Autodesk Inventor part; units mm, degrees
(part 2 of 3)
sketch "Sketch6" plane through (0, 6405, 0) normal (0, 1, 0) x (1, 0, 0)
  line L0 (350, -424.749) -> (350, 440.76)
  arc A0 (24.4727, -474.749) -> (24.4727, -424.749) centre (24.4727, -449.749) ccw
  arc A1 (-24.4727, -424.749) -> (-24.4727, -474.749) centre (-24.4727, -449.749) ccw
  line L1 (-350, -424.749) -> (-350, 440.76)
  line L2 (335.0195, -474.749) -> (364.9805, -474.749)
  line L3 (335.0195, -424.749) -> (364.9805, -424.749)
  arc A2 (364.9805, -474.749) -> (364.9805, -424.749) centre (364.9805, -449.749) ccw
  arc A3 (335.0195, -424.749) -> (335.0195, -474.749) centre (335.0195, -449.749) ccw
  line L4 (0, -424.749) -> (0, 440.76)
  line L5 (-24.4727, -474.749) -> (24.4727, -474.749)
  line L6 (-24.4727, -424.749) -> (24.4727, -424.749)
  line L7 (-364.9805, -474.749) -> (-335.0195, -474.749)
  line L8 (-489.5054, 350) -> (407.7236, 350)
  line L9 (-544.4663, 325) -> (-514.5054, 325)
  line L10 (-544.4663, 375) -> (-514.5054, 375)
  arc A4 (-514.5054, 325) -> (-514.5054, 375) centre (-514.5054, 350) ccw
  arc A5 (-544.4663, 375) -> (-544.4663, 325) centre (-544.4663, 350) ccw
  line L11 (-489.5054, 0) -> (-476.6036, 0)
  line L12 (-441.6036, 0) -> (407.7236, 0)
  line L13 (-559.9204, -25) -> (-514.5054, -25)
  line L14 (-559.9204, 25) -> (-514.5054, 25)
  arc A6 (-514.5054, -25) -> (-514.5054, 25) centre (-514.5054, 0) ccw
  line L15 (-364.9805, -424.749) -> (-335.0195, -424.749)
  arc A7 (-335.0195, -474.749) -> (-335.0195, -424.749) centre (-335.0195, -449.749) ccw
  arc A8 (-364.9805, -424.749) -> (-364.9805, -474.749) centre (-364.9805, -449.749) ccw
  line L16 (-489.5054, -350) -> (407.7236, -350)
  line L17 (-544.4663, -375) -> (-514.5054, -375)
  line L18 (-544.4663, -325) -> (-514.5054, -325)
  arc A9 (-514.5054, -375) -> (-514.5054, -325) centre (-514.5054, -350) ccw
  arc A10 (-544.4663, -325) -> (-544.4663, -375) centre (-544.4663, -350) ccw
  line L19 (145.0003, 447.2664) -> (120.0003, 442.2664)
  line L20 (120.0003, 130.0003) -> (120.0003, 467.2664)
  line L21 (120.0003, 442.2664) -> (350, 442.2664)
  line L22 (-439.1036, 145.0003) -> (-429.1036, 145.0003)
  line L23 (-429.1036, 145.0003) -> (-434.1036, 120.0003)
  line L24 (-439.1036, 145.0003) -> (-434.1036, 120.0003)
  line L25 (-130.0003, 120.0003) -> (-459.1036, 120.0003)
  line L26 (-434.1036, 120.0003) -> (-434.1036, 350)
  line L27 (-145.0003, 437.2664) -> (-145.0003, 447.2664)
  line L28 (-145.0003, 447.2664) -> (-120.0003, 442.2664)
  line L29 (-145.0003, 437.2664) -> (-120.0003, 442.2664)
  line L30 (-120.0003, 130.0003) -> (-120.0003, 467.2664)
  line L31 (-325, 447.2664) -> (-325, 437.2664)
  line L32 (-325, 437.2664) -> (-350, 442.2664)
  line L33 (-325, 447.2664) -> (-350, 442.2664)
  line L34 (-439.1036, -95.0003) -> (-434.1036, -120.0003)
  line L35 (-350, 360) -> (-350, 467.2664)
  line L36 (-350, 442.2664) -> (-120.0003, 442.2664)
  line L37 (95.0003, 437.2664) -> (95.0003, 447.2664)
  line L38 (95.0003, 447.2664) -> (120.0003, 442.2664)
  line L39 (95.0003, 437.2664) -> (120.0003, 442.2664)
  line L40 (120.0003, 130.0003) -> (120.0003, 467.2664)
  line L41 (-95.0003, 447.2664) -> (-95.0003, 437.2664)
  line L42 (-95.0003, 437.2664) -> (-120.0003, 442.2664)
  line L43 (-95.0003, 447.2664) -> (-120.0003, 442.2664)
  line L44 (-120.0003, 130.0003) -> (-120.0003, 467.2664)
  line L45 (-120.0003, 442.2664) -> (120.0003, 442.2664)
  line L46 (325, 437.2664) -> (325, 447.2664)
  line L47 (325, 447.2664) -> (350, 442.2664)
  line L48 (325, 437.2664) -> (350, 442.2664)
  line L49 (350, 360) -> (350, 467.2664)
  line L50 (145.0003, 447.2664) -> (145.0003, 437.2664)
  line L51 (145.0003, 437.2664) -> (120.0003, 442.2664)
  line L52 (350, 442.2664) -> (646.147, 442.2664)
  line L53 (-360, 350) -> (-459.1036, 350)
  line L54 (-429.1036, 325) -> (-434.1036, 350)
  line L55 (-439.1036, 325) -> (-434.1036, 350)
  line L56 (-429.1036, 325) -> (-439.1036, 325)
  line L57 (-434.1036, -120.0003) -> (-434.1036, 120.0003)
  line L58 (-130.0003, -120.0003) -> (-459.1036, -120.0003)
  line L59 (-429.1036, -95.0003) -> (-434.1036, -120.0003)
  line L60 (-439.1036, -95.0003) -> (-429.1036, -95.0003)
  line L61 (-130.0003, 120.0003) -> (-459.1036, 120.0003)
  line L62 (-429.1036, 95.0003) -> (-434.1036, 120.0003)
  line L63 (-439.1036, 95.0003) -> (-434.1036, 120.0003)
  line L64 (-429.1036, 95.0003) -> (-439.1036, 95.0003)
  line L65 (-434.1036, -350) -> (-434.1036, -120.0003)
  line L66 (-360, -350) -> (-459.1036, -350)
  line L67 (-439.1036, -325) -> (-434.1036, -350)
  line L68 (-429.1036, -325) -> (-434.1036, -350)
  line L69 (-439.1036, -325) -> (-429.1036, -325)
  line L70 (-130.0003, -120.0003) -> (-459.1036, -120.0003)
  line L71 (-429.1036, -145.0003) -> (-434.1036, -120.0003)
  line L72 (-439.1036, -145.0003) -> (-434.1036, -120.0003)
  line L73 (-429.1036, -145.0003) -> (-439.1036, -145.0003)
  line L74 (-350, 310) -> (-350, 350)
  line L75 (-342, 318) -> (-342, 332)
  line L76 (-318, 342) -> (-332, 342)
  line L77 (-310, 350) -> (-350, 350)
  line L78 (-342, 332) -> (-341.2388, 335.8268)
  arc A11 (-335.8268, 341.2388) -> (-341.2388, 335.8268) centre (-332, 332) ccw
  line L79 (-335.8268, 341.2388) -> (-332, 342)
  line L80 (-318, -342) -> (-332, -342)
  line L81 (-342, -332) -> (-342, -318)
  line L82 (-350, -350) -> (-350, -310)
  line L83 (-310, -350) -> (-350, -350)
  line L84 (-332, -342) -> (-335.8268, -341.2388)
  arc A12 (-341.2388, -335.8268) -> (-335.8268, -341.2388) centre (-332, -332) ccw
  line L85 (-341.2388, -335.8268) -> (-342, -332)
  line L86 (350, -350) -> (350, -310)
  line L87 (342, -332) -> (342, -318)
  line L88 (332, -342) -> (318, -342)
  line L89 (350, -350) -> (310, -350)
  line L90 (342, -332) -> (341.2388, -335.8268)
  arc A13 (335.8268, -341.2388) -> (341.2388, -335.8268) centre (332, -332) ccw
  line L91 (335.8268, -341.2388) -> (332, -342)
  circle A14 centre (-120, -120) radius 9
  line L92 (-102, -120) -> (-138, -120)
  line L93 (-120, -102) -> (-120, -138)
  circle A15 centre (120, -120) radius 9
  line L94 (138, -120) -> (102, -120)
  line L95 (120, -102) -> (120, -138)
  circle A16 centre (-120, 120) radius 9
  line L96 (-102, 120) -> (-138, 120)
  line L97 (-120, 138) -> (-120, 102)
  circle A17 centre (120, 120) radius 9
  line L98 (138, 120) -> (102, 120)
  line L99 (120, 138) -> (120, 102)
  line L100 (-354, 0) -> (-342, 0)
  line L101 (-350, 4) -> (-342, 4)
  line L102 (-350, -4) -> (-342, -4)
  line L103 (350, 310) -> (310, 350)
  line L104 (310, 350) -> (-310, 350)
  line L105 (350, 310) -> (350, -310)
  line L106 (350, -310) -> (310, -350)
  line L107 (-310, -350) -> (-350, -310)
  line L108 (-350, -310) -> (-350, 310)
  line L109 (-350, 310) -> (-310, 350)
  line L110 (310, -350) -> (-310, -350)
  line L111 (332, 342) -> (318, 342)
  line L112 (342, 318) -> (342, 332)
  line L113 (350, 310) -> (350, 350)
  line L114 (350, 350) -> (310, 350)
  line L115 (332, 342) -> (335.8268, 341.2388)
  arc A18 (341.2388, 335.8268) -> (335.8268, 341.2388) centre (332, 332) ccw
  line L116 (341.2388, 335.8268) -> (342, 332)
  line L117 (-347, 270) -> (-345.0866, 270.3806)
  line L118 (273.0866, -342.3806) -> (271.4645, -343.4645)
  line L119 (271.4645, -343.4645) -> (270.3806, -345.0866)
  line L120 (-270.3806, 345.0866) -> (-270, 347)
  line L121 (-271.4645, 343.4645) -> (-270.3806, 345.0866)
  line L122 (-273.0866, 342.3806) -> (-271.4645, 343.4645)
  line L123 (-275, 342) -> (-273.0866, 342.3806)
  line L124 (-342.3806, 273.0866) -> (-342, 275)
  line L125 (-343.4645, 271.4645) -> (-342.3806, 273.0866)
  line L126 (-345.0866, 270.3806) -> (-343.4645, 271.4645)
  line L127 (342, 275) -> (342.3806, 273.0866)
  line L128 (-270, 350) -> (-310, 350)
  line L129 (-270, 347) -> (-270, 350)
  line L130 (-275, 342) -> (-318, 342)
  line L131 (-342, 275) -> (-342, 318)
  line L132 (-350, 270) -> (-347, 270)
  line L133 (-350, 270) -> (-350, 310)
  line L134 (345.0866, 270.3806) -> (347, 270)
  line L135 (343.4645, 271.4645) -> (345.0866, 270.3806)
  line L136 (342.3806, 273.0866) -> (343.4645, 271.4645)
  line L137 (270.3806, -345.0866) -> (270, -347)
  line L138 (273.0866, 342.3806) -> (275, 342)
  line L139 (271.4645, 343.4645) -> (273.0866, 342.3806)
  line L140 (270.3806, 345.0866) -> (271.4645, 343.4645)
  line L141 (270, 347) -> (270.3806, 345.0866)
  line L142 (310, 350) -> (270, 350)
  line L143 (350, 270) -> (350, 310)
  line L144 (347, 270) -> (350, 270)
  line L145 (342, 275) -> (342, 318)
  line L146 (318, 342) -> (275, 342)
  line L147 (270, 347) -> (270, 350)
  line L148 (342, 270) -> (350, 270)
  line L149 (342, -270) -> (342, 270)
  line L150 (350, -270) -> (342, -270)
  line L151 (270, 342) -> (270, 350)
  line L152 (-270, 342) -> (270, 342)
  line L153 (-270, 350) -> (-270, 342)
  line L154 (270, 350) -> (-270, 350)
  line L155 (-342, 270) -> (-350, 270)
  line L156 (-342, -270) -> (-342, 270)
  line L157 (-350, -270) -> (-342, -270)
  line L158 (-350, 270) -> (-350, -270)
  line L159 (-270, -342) -> (270, -342)
  line L160 (-270, -350) -> (-270, -342)
  line L161 (270, -350) -> (270, -342)
  line L162 (-270, -350) -> (270, -350)
  line L163 (-270.3806, -345.0866) -> (-271.4645, -343.4645)
  line L164 (-271.4645, -343.4645) -> (-273.0866, -342.3806)
  line L165 (-273.0866, -342.3806) -> (-275, -342)
  line L166 (-342, -275) -> (-342.3806, -273.0866)
  line L167 (-342.3806, -273.0866) -> (-343.4645, -271.4645)
  line L168 (-343.4645, -271.4645) -> (-345.0866, -270.3806)
  line L169 (-345.0866, -270.3806) -> (-347, -270)
  line L170 (-270, -350) -> (-270, -347)
  line L171 (-275, -342) -> (-318, -342)
  line L172 (350, 270) -> (350, -270)
  line L173 (-342, -318) -> (-342, -275)
  line L174 (-350, -270) -> (-347, -270)
  line L175 (-350, -310) -> (-350, -270)
  line L176 (-270, -350) -> (-310, -350)
  line L177 (-270, -347) -> (-270.3806, -345.0866)
  line L178 (350, -310) -> (350, -270)
  line L179 (350, -270) -> (347, -270)
  line L180 (342, -318) -> (342, -275)
  line L181 (318, -342) -> (275, -342)
  line L182 (270, -350) -> (270, -347)
  line L183 (310, -350) -> (270, -350)
  line L184 (347, -270) -> (345.0866, -270.3806)
  line L185 (345.0866, -270.3806) -> (343.4645, -271.4645)
  line L186 (343.4645, -271.4645) -> (342.3806, -273.0866)
  line L187 (342.3806, -273.0866) -> (342, -275)
  line L188 (275, -342) -> (273.0866, -342.3806)
  line L189 (379.0739, 240.3123) -> (409.0739, 240.3123)
  line L190 (409.0739, 215.6456) -> (605.1413, 215.6456)
  line L191 (409.0739, 252.6456) -> (605.1413, 252.6456)
  line L192 (605.1413, 215.6456) -> (605.1413, 252.6456)
  line L193 (409.0739, 215.6456) -> (409.0739, 252.6456)
  line L194 (120, 120) -> (379.0739, 240.3123)
  line L195 (-58.2993, 546.2236) -> (67.1733, 546.2236)
  point P0 (0, 0)
  point P1 (-354.9805, -464.749)
  point P2 (-14.4727, -464.749)
  point P3 (345.0195, -464.749)
  point P4 (-534.4663, 335)
  point P5 (-549.9204, -15)
  point P6 (-534.4663, -365)
  point P7 (-262.8139, 454.7664)
  point P8 (375, 454.7664)
  point P9 (-27.8137, 454.7664)
  point P10 (207.1864, 454.7664)
  point P11 (-446.6036, 207.1864)
  point P12 (-446.6036, -27.8137)
  point P13 (-446.6036, -262.8139)
  point P14 (415.0739, 221.6456)
  point P15 (442.9231, 221.6456)
  point P16 (537.1784, 221.6456)
  point P17 (21.5405, 553.7236)
  point P18 (-25.7205, 513.7236)
  point P19 (-12.6665, 553.7236)
  point P20 (-58.2993, 553.7236)
  constraints: 384 end point, 47 point on line, 33 point on circle, 19 centre point, 4 midpoint, 66 other
sketch "Sketch7" plane through (0, 6405, 0) normal (0, 1, 0) x (1, 0, 0)
  line L0 (-350, -350) -> (-270, -350) projected
  line L1 (-310, -350) -> (-350, -310)
  line L2 (-350, -270) -> (-350, -350) projected
  line L3 (-350, -310) -> (-350, 310)
  line L4 (-350, 350) -> (-350, 270) projected
  line L5 (-350, 310) -> (-310, 350)
  line L6 (-310, 350) -> (310, 350)
  line L7 (310, 350) -> (350, 310)
  line L8 (350, 310) -> (350, -310)
  line L9 (350, -310) -> (310, -350)
  line L10 (310, -350) -> (-310, -350)
  circle A0 centre (-120, -120) radius 9 projected
  circle A1 centre (120, -120) radius 9 projected
  circle A2 centre (120, 120) radius 9 projected
  circle A3 centre (-120, 120) radius 9 projected
  point P0 (0, 0)
  constraints: 16 end point, 4 perpendicular, 3 midpoint, 1 collinear, 1 parallel
extrude "Extrusion17" add sketch "Sketch7" along normal blind 10 separate body contours L1 L2 L3 L5 L6 L7 L8 L9 L10 L0
sketch "Sketch8" plane through (-270, 15, 350) normal (0, 0, 1) x (1, 0, 0)
  arc A0 (33330.0195, 14726.87) -> (33330.0195, 14676.87) centre (33330.0195, 14701.87) ccw
  arc A1 (34059.9805, 14676.87) -> (34059.9805, 14726.87) centre (34059.9805, 14701.87) ccw
  arc A2 (34030.0195, 14726.87) -> (34030.0195, 14676.87) centre (34030.0195, 14701.87) ccw
  line L0 (33695, 14726.87) -> (33695, 15412.2236)
  line L1 (33695, 15461.2236) -> (33695, 21400.56)
  line L2 (33672.2925, 14676.87) -> (33717.7075, 14676.87)
  line L3 (33672.2925, 14726.87) -> (33717.7075, 14726.87)
  arc A3 (33717.7075, 14676.87) -> (33717.7075, 14726.87) centre (33717.7075, 14701.87) ccw
  arc A4 (33672.2925, 14726.87) -> (33672.2925, 14676.87) centre (33672.2925, 14701.87) ccw
  line L4 (33345, 14726.87) -> (33345, 21400.56)
  line L5 (33330.0195, 14676.87) -> (33359.9805, 14676.87)
  line L6 (33187.65, 14882.4) -> (34188.23, 14882.4)
  line L7 (33040.2135, 14857.4) -> (33162.65, 14857.4)
  line L8 (33040.2135, 14907.4) -> (33162.65, 14907.4)
  arc A5 (33162.65, 14857.4) -> (33162.65, 14907.4) centre (33162.65, 14882.4) ccw
  line L9 (33330.0195, 14726.87) -> (33359.9805, 14726.87)
  arc A6 (33040.2135, 14907.4) -> (33040.2135, 14857.4) centre (33040.2135, 14882.4) ccw
  line L10 (34045, 14726.87) -> (34045, 15229.9)
  line L11 (33187.65, 21282.4) -> (34188.23, 21282.4)
  line L12 (34045, 15264.9) -> (34045, 21400.56)
  line L13 (34030.0195, 14676.87) -> (34059.9805, 14676.87)
  line L14 (34030.0195, 14726.87) -> (34059.9805, 14726.87)
  line L15 (33025.7555, 21257.4) -> (33162.65, 21257.4)
  line L16 (33025.7555, 21307.4) -> (33162.65, 21307.4)
  arc A7 (33162.65, 21257.4) -> (33162.65, 21307.4) centre (33162.65, 21282.4) ccw
  arc A8 (33025.7555, 21307.4) -> (33025.7555, 21257.4) centre (33025.7555, 21282.4) ccw
  arc A9 (33359.9805, 14676.87) -> (33359.9805, 14726.87) centre (33359.9805, 14701.87) ccw
  arc A10 (34483.8578, 21307.4) -> (34483.8578, 21257.4) centre (34483.8578, 21282.4) ccw
  arc A11 (34498.3158, 14907.4) -> (34498.3158, 14857.4) centre (34498.3158, 14882.4) ccw
  line L17 (34320.5776, 17577.4) -> (34310.5776, 17577.4)
  line L18 (34310.5776, 17577.4) -> (34315.5776, 17602.4)
  line L19 (34320.5776, 17577.4) -> (34315.5776, 17602.4)
  line L20 (34315.5776, 19702.4) -> (34315.5776, 20052.4)
  line L21 (34320.5776, 16177.4) -> (34310.5776, 16177.4)
  line L22 (34310.5776, 16177.4) -> (34315.5776, 16202.4)
  line L23 (34320.5776, 16177.4) -> (34315.5776, 16202.4)
  line L24 (34015, 16202.4) -> (34335.5776, 16202.4)
  line L25 (34320.5776, 19677.4) -> (34310.5776, 19677.4)
  line L26 (34310.5776, 19677.4) -> (34315.5776, 19702.4)
  line L27 (34320.5776, 19677.4) -> (34315.5776, 19702.4)
  line L28 (34015, 19702.4) -> (34335.5776, 19702.4)
  line L29 (34310.5776, 19377.4) -> (34320.5776, 19377.4)
  line L30 (34320.5776, 19377.4) -> (34315.5776, 19352.4)
  line L31 (34015, 17602.4) -> (34335.5776, 17602.4)
  line L32 (34310.5776, 17277.4) -> (34320.5776, 17277.4)
  line L33 (34320.5776, 17277.4) -> (34315.5776, 17252.4)
  line L34 (34310.5776, 17277.4) -> (34315.5776, 17252.4)
  line L35 (34310.5776, 19377.4) -> (34315.5776, 19352.4)
  line L36 (34015, 19352.4) -> (34335.5776, 19352.4)
  line L37 (34315.5776, 19352.4) -> (34315.5776, 19702.4)
  line L38 (34320.5776, 19327.4) -> (34310.5776, 19327.4)
  line L39 (34310.5776, 19327.4) -> (34315.5776, 19352.4)
  line L40 (34015, 17252.4) -> (34335.5776, 17252.4)
  line L41 (34310.5776, 15877.4) -> (34320.5776, 15877.4)
  line L42 (34320.5776, 15877.4) -> (34315.5776, 15852.4)
  line L43 (34310.5776, 15877.4) -> (34315.5776, 15852.4)
  line L44 (34320.5776, 19327.4) -> (34315.5776, 19352.4)
  line L45 (34015, 19352.4) -> (34335.5776, 19352.4)
  line L46 (34310.5776, 19027.4) -> (34320.5776, 19027.4)
  line L47 (34320.5776, 19027.4) -> (34315.5776, 19002.4)
  line L48 (34310.5776, 19027.4) -> (34315.5776, 19002.4)
  line L49 (34015, 19002.4) -> (34335.5776, 19002.4)
  line L50 (34315.5776, 19002.4) -> (34315.5776, 19352.4)
  line L51 (34315.5776, 17252.4) -> (34315.5776, 17602.4)
  line L52 (34320.5776, 18977.4) -> (34310.5776, 18977.4)
  line L53 (34310.5776, 18977.4) -> (34315.5776, 19002.4)
  line L54 (34320.5776, 17227.4) -> (34310.5776, 17227.4)
  line L55 (34310.5776, 17227.4) -> (34315.5776, 17252.4)
  line L56 (34320.5776, 17227.4) -> (34315.5776, 17252.4)
  line L57 (34015, 15852.4) -> (34335.5776, 15852.4)
  line L58 (34315.5776, 15852.4) -> (34315.5776, 16202.4)
  line L59 (34015, 17252.4) -> (34335.5776, 17252.4)
  line L60 (34310.5776, 16927.4) -> (34320.5776, 16927.4)
  line L61 (34320.5776, 16927.4) -> (34315.5776, 16902.4)
  line L62 (34310.5776, 16927.4) -> (34315.5776, 16902.4)
  line L63 (34015, 16902.4) -> (34335.5776, 16902.4)
  line L64 (34315.5776, 16902.4) -> (34315.5776, 17252.4)
  line L65 (34320.5776, 15827.4) -> (34310.5776, 15827.4)
  line L66 (34015, 17952.4) -> (34335.5776, 17952.4)
  line L67 (34310.5776, 15827.4) -> (34315.5776, 15852.4)
  line L68 (34320.5776, 16877.4) -> (34310.5776, 16877.4)
  line L69 (34310.5776, 16877.4) -> (34315.5776, 16902.4)
  line L70 (34320.5776, 16877.4) -> (34315.5776, 16902.4)
  line L71 (34320.5776, 20377.4) -> (34315.5776, 20402.4)
  line L72 (34015, 16902.4) -> (34335.5776, 16902.4)
  line L73 (34310.5776, 16577.4) -> (34320.5776, 16577.4)
  line L74 (34320.5776, 16577.4) -> (34315.5776, 16552.4)
  line L75 (34310.5776, 16577.4) -> (34315.5776, 16552.4)
  line L76 (34320.5776, 15827.4) -> (34315.5776, 15852.4)
  line L77 (34015, 15852.4) -> (34335.5776, 15852.4)
  line L78 (34310.5776, 15527.4) -> (34320.5776, 15527.4)
  line L79 (34320.5776, 15527.4) -> (34315.5776, 15502.4)
  line L80 (34015, 16552.4) -> (34335.5776, 16552.4)
  line L81 (34315.5776, 16552.4) -> (34315.5776, 16902.4)
  line L82 (34310.5776, 15527.4) -> (34315.5776, 15502.4)
  line L83 (34015, 15502.4) -> (34335.5776, 15502.4)
  line L84 (34315.5776, 15502.4) -> (34315.5776, 15852.4)
  line L85 (34315.5776, 14882.4) -> (34315.5776, 15502.4)
  line L86 (34055, 14882.4) -> (34335.5776, 14882.4)
  line L87 (34310.5776, 14907.4) -> (34315.5776, 14882.4)
  line L88 (34320.5776, 14907.4) -> (34315.5776, 14882.4)
  line L89 (34310.5776, 14907.4) -> (34320.5776, 14907.4)
  line L90 (34015, 15502.4) -> (34335.5776, 15502.4)
  line L91 (34320.5776, 18977.4) -> (34315.5776, 19002.4)
  line L92 (34015, 19002.4) -> (34335.5776, 19002.4)
  line L93 (34310.5776, 18677.4) -> (34320.5776, 18677.4)
  line L94 (34320.5776, 18677.4) -> (34315.5776, 18652.4)
  line L95 (34320.5776, 15477.4) -> (34315.5776, 15502.4)
  line L96 (34310.5776, 15477.4) -> (34315.5776, 15502.4)
  line L97 (34320.5776, 15477.4) -> (34310.5776, 15477.4)
  line L98 (34310.5776, 18677.4) -> (34315.5776, 18652.4)
  line L99 (34015, 18652.4) -> (34335.5776, 18652.4)
  line L100 (34315.5776, 18652.4) -> (34315.5776, 19002.4)
  line L101 (34320.5776, 18627.4) -> (34310.5776, 18627.4)
  line L102 (34310.5776, 18627.4) -> (34315.5776, 18652.4)
  line L103 (34320.5776, 18627.4) -> (34315.5776, 18652.4)
  line L104 (34015, 18652.4) -> (34335.5776, 18652.4)
  line L105 (34310.5776, 18327.4) -> (34320.5776, 18327.4)
  line L106 (34320.5776, 18327.4) -> (34315.5776, 18302.4)
  line L107 (34310.5776, 18327.4) -> (34315.5776, 18302.4)
  line L108 (34015, 18302.4) -> (34335.5776, 18302.4)
  line L109 (34315.5776, 18302.4) -> (34315.5776, 18652.4)
  line L110 (34320.5776, 18277.4) -> (34310.5776, 18277.4)
  line L111 (34310.5776, 18277.4) -> (34315.5776, 18302.4)
  line L112 (34320.5776, 18277.4) -> (34315.5776, 18302.4)
  line L113 (34015, 18302.4) -> (34335.5776, 18302.4)
  line L114 (34310.5776, 17977.4) -> (34320.5776, 17977.4)
  line L115 (34320.5776, 17977.4) -> (34315.5776, 17952.4)
  line L116 (34310.5776, 17977.4) -> (34315.5776, 17952.4)
  line L117 (34015, 17952.4) -> (34335.5776, 17952.4)
  line L118 (34320.5776, 19727.4) -> (34315.5776, 19702.4)
  line L119 (34315.5776, 17952.4) -> (34315.5776, 18302.4)
  line L120 (34315.5776, 14882.4) -> (34315.5776, 14686.3019)
  line L121 (34206.209, 14882.4) -> (34206.209, 15152.4)
  line L122 (34065, 14882.4) -> (34226.209, 14882.4)
  line L123 (34201.209, 14907.4) -> (34206.209, 14882.4)
  line L124 (34211.209, 14907.4) -> (34206.209, 14882.4)
  line L125 (34201.209, 14907.4) -> (34211.209, 14907.4)
  line L126 (34015.0003, 15152.4) -> (34226.209, 15152.4)
  line L127 (34211.209, 15127.4) -> (34206.209, 15152.4)
  line L128 (34201.209, 15127.4) -> (34206.209, 15152.4)
  line L129 (34211.209, 15127.4) -> (34201.209, 15127.4)
  line L130 (34206.209, 14882.4) -> (34206.209, 14651.0602)
  line L131 (34320.5776, 16527.4) -> (34310.5776, 16527.4)
  line L132 (34310.5776, 16527.4) -> (34315.5776, 16552.4)
  line L133 (34320.5776, 16527.4) -> (34315.5776, 16552.4)
  line L134 (34015, 16552.4) -> (34335.5776, 16552.4)
  line L135 (34310.5776, 16227.4) -> (34320.5776, 16227.4)
  line L136 (34320.5776, 16227.4) -> (34315.5776, 16202.4)
  line L137 (34320.5776, 17927.4) -> (34310.5776, 17927.4)
  line L138 (34310.5776, 17927.4) -> (34315.5776, 17952.4)
  line L139 (34320.5776, 17927.4) -> (34315.5776, 17952.4)
  line L140 (34310.5776, 17627.4) -> (34320.5776, 17627.4)
  line L141 (34320.5776, 17627.4) -> (34315.5776, 17602.4)
  line L142 (34310.5776, 17627.4) -> (34315.5776, 17602.4)
  line L143 (34015, 17602.4) -> (34335.5776, 17602.4)
  line L144 (34315.5776, 17602.4) -> (34315.5776, 17952.4)
  line L145 (34310.5776, 16227.4) -> (34315.5776, 16202.4)
  line L146 (34015, 16202.4) -> (34335.5776, 16202.4)
  line L147 (34315.5776, 16202.4) -> (34315.5776, 16552.4)
  line L148 (34310.5776, 19727.4) -> (34320.5776, 19727.4)
  line L149 (34015, 20052.4) -> (34335.5776, 20052.4)
  line L150 (34320.5776, 20027.4) -> (34315.5776, 20052.4)
  line L151 (34310.5776, 20027.4) -> (34315.5776, 20052.4)
  line L152 (34320.5776, 20027.4) -> (34310.5776, 20027.4)
  line L153 (34315.5776, 20052.4) -> (34315.5776, 20402.4)
  line L154 (34015, 20052.4) -> (34335.5776, 20052.4)
  line L155 (34310.5776, 20077.4) -> (34315.5776, 20052.4)
  line L156 (34320.5776, 20077.4) -> (34315.5776, 20052.4)
  line L157 (34310.5776, 20077.4) -> (34320.5776, 20077.4)
  line L158 (34015, 20402.4) -> (34047, 20402.4)
  line L159 (34082, 20402.4) -> (34335.5776, 20402.4)
  line L160 (34310.5776, 19727.4) -> (34315.5776, 19702.4)
  line L161 (34310.5776, 20377.4) -> (34315.5776, 20402.4)
  line L162 (34320.5776, 20377.4) -> (34310.5776, 20377.4)
  line L163 (34315.5776, 20402.4) -> (34315.5776, 20752.4)
  line L164 (34015, 20402.4) -> (34047, 20402.4)
  line L165 (34082, 20402.4) -> (34335.5776, 20402.4)
  line L166 (34310.5776, 20427.4) -> (34315.5776, 20402.4)
  line L167 (34320.5776, 20427.4) -> (34315.5776, 20402.4)
  line L168 (34310.5776, 20427.4) -> (34320.5776, 20427.4)
  line L169 (34015, 20752.4) -> (34335.5776, 20752.4)
  line L170 (34320.5776, 20727.4) -> (34315.5776, 20752.4)
  line L171 (34310.5776, 20727.4) -> (34315.5776, 20752.4)
  line L172 (34320.5776, 20727.4) -> (34310.5776, 20727.4)
  line L173 (34315.5776, 20752.4) -> (34315.5776, 21102.4)
  line L174 (34015, 20752.4) -> (34335.5776, 20752.4)
  line L175 (34310.5776, 20777.4) -> (34315.5776, 20752.4)
  line L176 (34320.5776, 20777.4) -> (34315.5776, 20752.4)
  line L177 (34310.5776, 20777.4) -> (34320.5776, 20777.4)
  line L178 (34015, 21102.4) -> (34335.5776, 21102.4)
  line L179 (34320.5776, 21077.4) -> (34315.5776, 21102.4)
  line L180 (34310.5776, 21077.4) -> (34315.5776, 21102.4)
  line L181 (34320.5776, 21077.4) -> (34310.5776, 21077.4)
  line L182 (34315.5776, 21102.4) -> (34315.5776, 21282.4)
  line L183 (34015, 21102.4) -> (34335.5776, 21102.4)
  line L184 (34310.5776, 21127.4) -> (34315.5776, 21102.4)
  line L185 (34320.5776, 21127.4) -> (34315.5776, 21102.4)
  line L186 (34310.5776, 21127.4) -> (34320.5776, 21127.4)
  line L187 (34055, 21282.4) -> (34335.5776, 21282.4)
  line L188 (34320.5776, 21257.4) -> (34315.5776, 21282.4)
  line L189 (34310.5776, 21257.4) -> (34315.5776, 21282.4)
  line L190 (34320.5776, 21257.4) -> (34310.5776, 21257.4)
  line L191 (33345, 21374.3106) -> (33695.0003, 21374.3106)
  line L192 (33345, 21292.4) -> (33345, 21399.3106)
  line L193 (33370, 21379.3106) -> (33345, 21374.3106)
  line L194 (33370, 21369.3106) -> (33345, 21374.3106)
  line L195 (33370, 21379.3106) -> (33370, 21369.3106)
  line L196 (33695.0003, 21232.3997) -> (33695.0003, 21399.3106)
  line L197 (33670.0003, 21369.3106) -> (33695.0003, 21374.3106)
  line L198 (33670.0003, 21379.3106) -> (33695.0003, 21374.3106)
  line L199 (33670.0003, 21369.3106) -> (33670.0003, 21379.3106)
  line L200 (33345, 21374.3106) -> (33187.8179, 21374.3106)
  line L201 (33695.0003, 21374.3106) -> (34045, 21374.3106)
  line L202 (33695.0003, 21232.3997) -> (33695.0003, 21399.3106)
  line L203 (33720.0003, 21379.3106) -> (33695.0003, 21374.3106)
  line L204 (33720.0003, 21369.3106) -> (33695.0003, 21374.3106)
  line L205 (33720.0003, 21379.3106) -> (33720.0003, 21369.3106)
  line L206 (34045, 21292.4) -> (34045, 21399.3106)
  line L207 (34020, 21369.3106) -> (34045, 21374.3106)
  line L208 (34020, 21379.3106) -> (34045, 21374.3106)
  line L209 (34020, 21369.3106) -> (34020, 21379.3106)
  line L210 (34134.4714, 21172.4) -> (34134.4714, 21222.3997)
  line L211 (33975, 21172.4) -> (34154.4714, 21172.4)
  line L212 (34139.4714, 21147.4) -> (34134.4714, 21172.4)
  line L213 (34129.4714, 21147.4) -> (34134.4714, 21172.4)
  line L214 (34139.4714, 21147.4) -> (34129.4714, 21147.4)
  line L215 (33705.0003, 21222.3997) -> (34154.4714, 21222.3997)
  line L216 (34129.4714, 21247.3997) -> (34134.4714, 21222.3997)
  line L217 (34139.4714, 21247.3997) -> (34134.4714, 21222.3997)
  line L218 (34129.4714, 21247.3997) -> (34139.4714, 21247.3997)
  line L219 (34134.4714, 21172.4) -> (34134.4714, 21147.4)
  line L220 (34134.4714, 21222.3997) -> (34134.4714, 21247.3997)
  line L221 (34134.4714, 21222.3997) -> (34134.4714, 21272.4)
  line L222 (33705.0003, 21222.3997) -> (34154.4714, 21222.3997)
  line L223 (34139.4714, 21247.3997) -> (34134.4714, 21222.3997)
  line L224 (34129.4714, 21247.3997) -> (34139.4714, 21247.3997)
  line L225 (33975, 21272.4) -> (34154.4714, 21272.4)
  line L226 (34139.4714, 21247.4) -> (34134.4714, 21272.4)
  line L227 (34129.4714, 21247.4) -> (34134.4714, 21272.4)
  line L228 (34139.4714, 21247.4) -> (34129.4714, 21247.4)
  line L229 (34005.0003, 15222.4) -> (34045, 15222.4)
  line L230 (34005.0003, 15162.4) -> (34005.0003, 15247.4)
  line L231 (33980.0003, 15217.4) -> (34005.0003, 15222.4)
  line L232 (33980.0003, 15227.4) -> (34005.0003, 15222.4)
  line L233 (33980.0003, 15217.4) -> (33980.0003, 15227.4)
  line L234 (34045, 14992.4) -> (34045, 15247.4)
  line L235 (34070, 15227.4) -> (34045, 15222.4)
  line L236 (34070, 15217.4) -> (34045, 15222.4)
  line L237 (34070, 15227.4) -> (34070, 15217.4)
  line L238 (34005.0003, 15222.4) -> (33980.0003, 15222.4)
  line L239 (34045, 15222.4) -> (34070, 15222.4)
  line L240 (34015, 19702.4) -> (34335.5776, 19702.4)
  line L241 (34129.4714, 21247.3997) -> (34134.4714, 21222.3997)
  line L242 (33965, 18822.4) -> (33965, 18722.4)
  line L243 (33965, 18722.4) -> (33425, 18722.4)
  circle A12 centre (33695, 21222.4) radius 4
  line L244 (33695, 21214.4) -> (33695, 21230.4)
  line L245 (33703, 21222.4) -> (33687, 21222.4)
  line L246 (33997, 18652.4) -> (34013, 18652.4)
  line L247 (33425, 21172.4) -> (33425, 21272.4)
  line L248 (33425, 21272.4) -> (33965, 21272.4)
  line L249 (33965, 21272.4) -> (33965, 21172.4)
  line L250 (33965, 21172.4) -> (33425, 21172.4)
  line L251 (33345, 21282.4) -> (34045, 21282.4)
  line L252 (34045, 21282.4) -> (34045, 21272.4)
  line L253 (34005, 21272.4) -> (33385, 21272.4)
  line L254 (33345, 21272.4) -> (33345, 21282.4)
  line L255 (34005, 21272.4) -> (34005, 21282.4)
  line L256 (33385, 21272.4) -> (33385, 21282.4)
  line L257 (33425, 19362.4) -> (33425, 19462.4)
  line L258 (33425, 19462.4) -> (33965, 19462.4)
  line L259 (33965, 19462.4) -> (33965, 19362.4)
  line L260 (33965, 19362.4) -> (33425, 19362.4)
  line L261 (33425, 20002.4) -> (33425, 20102.4)
  line L262 (33425, 20102.4) -> (33965, 20102.4)
  line L263 (33965, 20102.4) -> (33965, 20002.4)
  line L264 (33965, 20002.4) -> (33425, 20002.4)
  line L265 (33425, 20642.4) -> (33425, 20742.4)
  line L266 (33425, 20742.4) -> (33965, 20742.4)
  line L267 (33965, 20742.4) -> (33965, 20642.4)
  line L268 (33965, 20642.4) -> (33425, 20642.4)
  circle A13 centre (34005, 15502.4) radius 4
  line L269 (34005, 15510.4) -> (34005, 15494.4)
  line L270 (33997, 15502.4) -> (34013, 15502.4)
  circle A14 centre (34005, 15852.4) radius 4
  line L271 (34005, 15860.4) -> (34005, 15844.4)
  line L272 (33997, 15852.4) -> (34013, 15852.4)
  circle A15 centre (34005, 16202.4) radius 4
  line L273 (34005, 16210.4) -> (34005, 16194.4)
  line L274 (33997, 16202.4) -> (34013, 16202.4)
  circle A16 centre (34005, 16552.4) radius 4
  line L275 (34005, 16560.4) -> (34005, 16544.4)
  line L276 (33997, 16552.4) -> (34013, 16552.4)
  circle A17 centre (34005, 16902.4) radius 4
  line L277 (34005, 16910.4) -> (34005, 16894.4)
  line L278 (33997, 16902.4) -> (34013, 16902.4)
  circle A18 centre (34005, 17252.4) radius 4
  line L279 (34005, 17260.4) -> (34005, 17244.4)
  line L280 (33997, 17252.4) -> (34013, 17252.4)
  circle A19 centre (34005, 17602.4) radius 4
  line L281 (34005, 17610.4) -> (34005, 17594.4)
  line L282 (33997, 17602.4) -> (34013, 17602.4)
  circle A20 centre (34005, 17952.4) radius 4
  line L283 (34005, 17960.4) -> (34005, 17944.4)
  line L284 (33997, 17952.4) -> (34013, 17952.4)
  circle A21 centre (34005, 18302.4) radius 4
  line L285 (34005, 18310.4) -> (34005, 18294.4)
  line L286 (33997, 18302.4) -> (34013, 18302.4)
  circle A22 centre (34005, 18652.4) radius 4
  line L287 (34005, 18660.4) -> (34005, 18644.4)
  circle A23 centre (34005, 19002.4) radius 4
  line L288 (34005, 19010.4) -> (34005, 18994.4)
  line L289 (33997, 19002.4) -> (34013, 19002.4)
  circle A24 centre (34005, 19352.4) radius 4
  line L290 (34005, 19360.4) -> (34005, 19344.4)
  line L291 (33997, 19352.4) -> (34013, 19352.4)
  circle A25 centre (34005, 19702.4) radius 4
  line L292 (34005, 19710.4) -> (34005, 19694.4)
  line L293 (33997, 19702.4) -> (34013, 19702.4)
  circle A26 centre (34005, 20052.4) radius 4
  line L294 (34005, 20060.4) -> (34005, 20044.4)
  line L295 (33997, 20052.4) -> (34013, 20052.4)
  circle A27 centre (34005, 20402.4) radius 4
  line L296 (34005, 20410.4) -> (34005, 20394.4)
  line L297 (33997, 20402.4) -> (34013, 20402.4)
  circle A28 centre (34005, 20752.4) radius 4
  line L298 (34005, 20760.4) -> (34005, 20744.4)
  line L299 (33997, 20752.4) -> (34013, 20752.4)
  circle A29 centre (34005, 21102.4) radius 4
  line L300 (34005, 21110.4) -> (34005, 21094.4)
  line L301 (33997, 21102.4) -> (34013, 21102.4)
  line L302 (33425, 16162.4) -> (33425, 16262.4)
  line L303 (33425, 16262.4) -> (33965, 16262.4)
  line L304 (33965, 16262.4) -> (33965, 16162.4)
  line L305 (33965, 16162.4) -> (33425, 16162.4)
  line L306 (33425, 16802.4) -> (33425, 16902.4)
  line L307 (33425, 16902.4) -> (33965, 16902.4)
  line L308 (33965, 16902.4) -> (33965, 16802.4)
  line L309 (33965, 16802.4) -> (33425, 16802.4)
  line L310 (33365, 14890.4) -> (33365, 14867.4)
  line L311 (33372, 14882.4) -> (33372, 14867.4)
  line L312 (33358, 14882.4) -> (33358, 14867.4)
  line L313 (34025, 14890.4) -> (34025, 14867.4)
  line L314 (34032, 14882.4) -> (34032, 14867.4)
  line L315 (34018, 14882.4) -> (34018, 14867.4)
  line L316 (33425, 14897.4) -> (33425, 14867.4)
  line L317 (33438, 14882.4) -> (33438, 14867.4)
  line L318 (33412, 14882.4) -> (33412, 14867.4)
  line L319 (33965, 14897.4) -> (33965, 14867.4)
  line L320 (33978, 14882.4) -> (33978, 14867.4)
  line L321 (33952, 14882.4) -> (33952, 14867.4)
  line L322 (34055, 14867.4) -> (34055, 14882.4)
  line L323 (34055, 14867.4) -> (33335, 14867.4)
  line L324 (34055, 14882.4) -> (33335, 14882.4)
  line L325 (33335, 14882.4) -> (33335, 14867.4)
  line L326 (34045, 14882.4) -> (34045, 15229.9)
  line L327 (34045, 15264.9) -> (34045, 21272.4)
  line L328 (33965, 21272.4) -> (33965, 14882.4)
  line L329 (34045, 21272.4) -> (33965, 21272.4)
  line L330 (33965, 18182.4) -> (33965, 18082.4)
  line L331 (33425, 21272.4) -> (33345, 21272.4)
  line L332 (33345, 21272.4) -> (33345, 14882.4)
  line L333 (33425, 14882.4) -> (33425, 21272.4)
  line L334 (33425, 15522.4) -> (33425, 15622.4)
  line L335 (33425, 15622.4) -> (33965, 15622.4)
  line L336 (33965, 15622.4) -> (33965, 15522.4)
  line L337 (33965, 15522.4) -> (33425, 15522.4)
  line L338 (33715, 14982.4) -> (33965, 14982.4)
  line L339 (33965, 14982.4) -> (33965, 14882.4)
  line L340 (33425, 14882.4) -> (33425, 14982.4)
  line L341 (33425, 14982.4) -> (33675, 14982.4)
  line L342 (33675, 14982.4) -> (33695, 14962.4)
  line L343 (33695, 14962.4) -> (33715, 14982.4)
  circle A30 centre (34005, 15152.4) radius 9
  line L344 (34005, 15170.4) -> (34005, 15134.4)
  line L345 (33987, 15152.4) -> (34023, 15152.4)
  line L346 (33425, 17442.4) -> (33425, 17542.4)
  line L347 (33425, 17542.4) -> (33965, 17542.4)
  line L348 (33965, 17542.4) -> (33965, 17442.4)
  line L349 (33965, 17442.4) -> (33425, 17442.4)
  line L350 (33425, 18082.4) -> (33425, 18182.4)
  line L351 (33425, 18182.4) -> (33965, 18182.4)
  line L352 (33965, 18082.4) -> (33425, 18082.4)
  line L353 (33425, 18722.4) -> (33425, 18822.4)
  line L354 (33425, 18822.4) -> (33965, 18822.4)
  line L355 (34037, 20742.4) -> (34037, 20642.4)
  line L356 (34045, 20742.4) -> (34037, 20742.4)
  line L357 (34045, 20642.4) -> (34045, 20742.4)
  line L358 (34037, 20642.4) -> (34045, 20642.4)
  line L359 (33353, 20002.4) -> (33353, 20102.4)
  line L360 (33345, 20002.4) -> (33353, 20002.4)
  line L361 (33345, 20102.4) -> (33345, 20002.4)
  line L362 (33353, 20102.4) -> (33345, 20102.4)
  line L363 (34037, 20102.4) -> (34037, 20002.4)
  line L364 (34045, 20102.4) -> (34037, 20102.4)
  line L365 (34045, 20002.4) -> (34045, 20102.4)
  line L366 (34037, 20002.4) -> (34045, 20002.4)
  line L367 (33353, 19362.4) -> (33353, 19462.4)
  line L368 (33345, 19362.4) -> (33353, 19362.4)
  line L369 (33345, 19462.4) -> (33345, 19362.4)
  line L370 (33353, 19462.4) -> (33345, 19462.4)
  line L371 (34037, 19462.4) -> (34037, 19362.4)
  line L372 (34045, 19462.4) -> (34037, 19462.4)
  line L373 (34045, 19362.4) -> (34045, 19462.4)
  line L374 (34037, 19362.4) -> (34045, 19362.4)
  line L375 (33385, 21272.4) -> (33345, 21272.4)
  line L376 (34045, 21272.4) -> (34005, 21272.4)
  line L377 (33353, 21172.4) -> (33353, 21272.4)
  line L378 (33345, 21172.4) -> (33353, 21172.4)
  line L379 (33345, 21272.4) -> (33345, 21172.4)
  line L380 (33353, 21272.4) -> (33345, 21272.4)
  line L381 (34037, 21272.4) -> (34037, 21172.4)
  line L382 (34045, 21272.4) -> (34037, 21272.4)
  line L383 (34045, 21172.4) -> (34045, 21272.4)
  line L384 (33345, 20742.4) -> (33345, 20642.4)
  line L385 (34037, 14982.4) -> (34037, 14882.4)
  line L386 (34045, 14982.4) -> (34037, 14982.4)
  line L387 (34045, 14882.4) -> (34045, 14982.4)
  line L388 (34037, 14882.4) -> (34045, 14882.4)
  line L389 (33965, 14882.4) -> (33425, 14882.4)
  line L390 (34037, 15622.4) -> (34037, 15522.4)
  line L391 (34045, 15622.4) -> (34037, 15622.4)
  line L392 (34045, 15522.4) -> (34045, 15622.4)
  line L393 (34037, 15522.4) -> (34045, 15522.4)
  line L394 (33353, 14882.4) -> (33353, 14982.4)
  line L395 (33345, 14882.4) -> (33353, 14882.4)
  line L396 (33345, 14982.4) -> (33345, 14882.4)
  line L397 (33353, 14982.4) -> (33345, 14982.4)
  line L398 (33353, 15522.4) -> (33353, 15622.4)
  line L399 (33345, 15522.4) -> (33353, 15522.4)
  line L400 (33345, 15622.4) -> (33345, 15522.4)
  line L401 (33353, 15622.4) -> (33345, 15622.4)
  line L402 (33353, 14882.4) -> (33353, 21272.4)
  line L403 (33345, 14882.4) -> (33425, 14882.4)
  line L404 (34037, 15229.9) -> (34037, 14882.4)
  line L405 (34037, 21272.4) -> (34037, 15264.9)
  line L406 (33965, 14882.4) -> (34045, 14882.4)
  line L407 (34037, 21172.4) -> (34045, 21172.4)
  line L408 (33353, 16802.4) -> (33353, 16902.4)
  line L409 (33345, 16802.4) -> (33353, 16802.4)
  line L410 (33345, 16902.4) -> (33345, 16802.4)
  line L411 (33353, 16902.4) -> (33345, 16902.4)
  line L412 (34037, 16902.4) -> (34037, 16802.4)
  line L413 (34045, 16902.4) -> (34037, 16902.4)
  line L414 (34045, 16802.4) -> (34045, 16902.4)
  line L415 (34037, 16802.4) -> (34045, 16802.4)
  line L416 (33353, 16162.4) -> (33353, 16262.4)
  line L417 (33345, 16162.4) -> (33353, 16162.4)
  line L418 (33345, 16262.4) -> (33345, 16162.4)
  line L419 (33353, 16262.4) -> (33345, 16262.4)
  line L420 (34037, 16262.4) -> (34037, 16162.4)
  line L421 (34045, 16262.4) -> (34037, 16262.4)
  line L422 (34045, 16162.4) -> (34045, 16262.4)
  line L423 (34037, 16162.4) -> (34045, 16162.4)
  line L424 (33353, 20642.4) -> (33353, 20742.4)
  line L425 (33353, 18722.4) -> (33353, 18822.4)
  line L426 (33345, 18722.4) -> (33353, 18722.4)
  line L427 (33345, 18822.4) -> (33345, 18722.4)
  line L428 (33353, 18822.4) -> (33345, 18822.4)
  line L429 (34037, 18822.4) -> (34037, 18722.4)
  line L430 (34045, 18822.4) -> (34037, 18822.4)
  line L431 (34045, 18722.4) -> (34045, 18822.4)
  line L432 (34037, 18722.4) -> (34045, 18722.4)
  line L433 (33353, 18082.4) -> (33353, 18182.4)
  line L434 (33345, 18082.4) -> (33353, 18082.4)
  line L435 (33345, 18182.4) -> (33345, 18082.4)
  line L436 (33353, 18182.4) -> (33345, 18182.4)
  line L437 (34037, 18182.4) -> (34037, 18082.4)
  line L438 (34045, 18182.4) -> (34037, 18182.4)
  line L439 (34045, 18082.4) -> (34045, 18182.4)
  line L440 (34037, 18082.4) -> (34045, 18082.4)
  line L441 (33353, 17442.4) -> (33353, 17542.4)
  line L442 (33345, 17442.4) -> (33353, 17442.4)
  line L443 (33345, 17542.4) -> (33345, 17442.4)
  line L444 (33353, 17542.4) -> (33345, 17542.4)
  line L445 (34037, 17542.4) -> (34037, 17442.4)
  line L446 (34045, 17542.4) -> (34037, 17542.4)
  line L447 (34045, 17442.4) -> (34045, 17542.4)
  line L448 (34037, 17442.4) -> (34045, 17442.4)
  line L449 (33345, 20642.4) -> (33353, 20642.4)
  line L450 (33353, 20742.4) -> (33345, 20742.4)
  line L451 (33759.3703, 15230.1871) -> (33880.9992, 15230.1871)
  line L452 (33759.3703, 15267.1871) -> (33880.9992, 15267.1871)
  line L453 (33880.9992, 15230.1871) -> (33880.9992, 15267.1871)
  line L454 (33759.3703, 15230.1871) -> (33759.3703, 15267.1871)
  line L455 (34004.9997, 15152.3997) -> (33910.9992, 15254.8538)
  line L456 (33910.9992, 15254.8538) -> (33880.9992, 15254.8538)
  line L457 (33215.4605, 14882.4) -> (33225.9606, 14917.4)
  line L458 (34148.7193, 14982.4) -> (34148.7193, 14882.4)
  line L459 (34159.2194, 14917.4) -> (34138.2194, 14917.4)
  line L460 (34171.4693, 14882.3999) -> (34113.7193, 14882.4001)
  line L461 (34148.7193, 14882.4) -> (34138.2194, 14917.4)
  line L462 (34148.7193, 14882.4) -> (34159.2194, 14917.4)
  line L463 (33215.4605, 14982.4) -> (33215.4605, 14882.4)
  line L464 (33215.4605, 14882.4) -> (33204.9606, 14917.4)
  line L465 (33766.061, 21111.5613) -> (33872.6875, 21111.5613)
  line L466 (33766.061, 21148.5613) -> (33872.6875, 21148.5613)
  line L467 (33872.6875, 21111.5613) -> (33872.6875, 21148.5613)
  line L468 (33766.061, 21111.5613) -> (33766.061, 21148.5613)
  line L469 (33696.2361, 21226.2042) -> (33736.061, 21136.2279)
  line L470 (33736.061, 21136.2279) -> (33766.061, 21136.2279)
  line L471 (33225.9606, 14917.4) -> (33204.9606, 14917.4)
  line L472 (33698.2155, 15418.2236) -> (33894.2828, 15418.2236)
  line L473 (33698.2155, 15455.2236) -> (33894.2828, 15455.2236)
  line L474 (33894.2828, 15418.2236) -> (33894.2828, 15455.2236)
  line L475 (33698.2155, 15418.2236) -> (33698.2155, 15455.2236)
  line L476 (34005, 15502.4) -> (33924.2828, 15442.8903)
  line L477 (33924.2828, 15442.8903) -> (33894.2828, 15442.8903)
  line L478 (33250.4605, 14882.3999) -> (33192.7105, 14882.4001)
  line L479 (33519.8539, 21486.9956) -> (33875.5961, 21486.9956)
  arc A31 (34046, 20387.3949) -> (34083, 20387.3949) centre (34064.5, 20387.3949) ccw
  arc A32 (34083, 20480.9623) -> (34046, 20480.9623) centre (34064.5, 20480.9623) ccw
  line L480 (34046, 20387.3949) -> (34046, 20480.9623)
  line L481 (34083, 20387.3949) -> (34083, 20480.9623)
  arc A33 (33477.5, 16300.4) -> (33477.5, 16263.4) centre (33477.5, 16281.9) ccw
  arc A34 (33580.2959, 16263.4) -> (33580.2959, 16300.4) centre (33580.2959, 16281.9) ccw
  line L482 (33477.5, 16300.4) -> (33580.2959, 16300.4)
  line L483 (33477.5, 16263.4) -> (33580.2959, 16263.4)
  arc A35 (33477.5, 16940.4) -> (33477.5, 16903.4) centre (33477.5, 16921.9) ccw
  arc A36 (33580.2959, 16903.4) -> (33580.2959, 16940.4) centre (33580.2959, 16921.9) ccw
  line L484 (33477.5, 16940.4) -> (33580.2959, 16940.4)
  line L485 (33477.5, 16903.4) -> (33580.2959, 16903.4)
  arc A37 (33274.5, 20331.9275) -> (33344, 20331.9275) centre (33309.25, 20331.9275) ccw
  arc A38 (33344, 20542.7899) -> (33274.5, 20542.7899) centre (33309.25, 20542.7899) ccw
  line L486 (33274.5, 20331.9275) -> (33274.5, 20542.7899)
  line L487 (33344, 20331.9275) -> (33344, 20542.7899)
  arc A39 (33468.2288, 15020.4) -> (33468.2288, 14983.4) centre (33468.2288, 15001.9) ccw
  arc A40 (33571.0247, 14983.4) -> (33571.0247, 15020.4) centre (33571.0247, 15001.9) ccw
  line L488 (33468.2288, 15020.4) -> (33571.0247, 15020.4)
  line L489 (33468.2288, 14983.4) -> (33571.0247, 14983.4)
  arc A41 (33468.2288, 15660.4) -> (33468.2288, 15623.4) centre (33468.2288, 15641.9) ccw
  arc A42 (33571.0247, 15623.4) -> (33571.0247, 15660.4) centre (33571.0247, 15641.9) ccw
  line L490 (33468.2288, 15660.4) -> (33571.0247, 15660.4)
  line L491 (33477.5, 20743.4) -> (33580.2959, 20743.4)
  line L492 (33477.5, 20780.4) -> (33580.2959, 20780.4)
  arc A43 (33580.2959, 20743.4) -> (33580.2959, 20780.4) centre (33580.2959, 20761.9) ccw
  arc A44 (33477.5, 20780.4) -> (33477.5, 20743.4) centre (33477.5, 20761.9) ccw
  line L493 (33477.5, 20103.4) -> (33580.2959, 20103.4)
  line L494 (33477.5, 20140.4) -> (33580.2959, 20140.4)
  arc A45 (33580.2959, 20103.4) -> (33580.2959, 20140.4) centre (33580.2959, 20121.9) ccw
  arc A46 (33477.5, 20140.4) -> (33477.5, 20103.4) centre (33477.5, 20121.9) ccw
  line L495 (33477.5, 19463.4) -> (33580.2959, 19463.4)
  line L496 (33477.5, 19500.4) -> (33580.2959, 19500.4)
  arc A47 (33580.2959, 19463.4) -> (33580.2959, 19500.4) centre (33580.2959, 19481.9) ccw
  arc A48 (33477.5, 19500.4) -> (33477.5, 19463.4) centre (33477.5, 19481.9) ccw
  line L497 (33393.529, 21291.4391) -> (33496.3249, 21291.4391)
  line L498 (33468.2288, 15623.4) -> (33571.0247, 15623.4)
  arc A49 (33496.3249, 21291.4391) -> (33496.3249, 21328.4391) centre (33496.3249, 21309.9391) ccw
  arc A50 (33393.529, 21328.4391) -> (33393.529, 21291.4391) centre (33393.529, 21309.9391) ccw
  line L499 (33365.245, 21281.6551) -> (33393.529, 21291.4391)
  line L500 (33558.294, 21130.894) -> (33661.0899, 21130.894)
  line L501 (33558.294, 21167.894) -> (33661.0899, 21167.894)
  arc A51 (33661.0899, 21130.894) -> (33661.0899, 21167.894) centre (33661.0899, 21149.394) ccw
  arc A52 (33558.294, 21167.894) -> (33558.294, 21130.894) centre (33558.294, 21149.394) ccw
  line L502 (33533.294, 21192.694) -> (33558.294, 21167.894)
  line L503 (33477.5, 18823.4) -> (33580.2959, 18823.4)
  line L504 (33477.5, 18860.4) -> (33580.2959, 18860.4)
  arc A53 (33580.2959, 18823.4) -> (33580.2959, 18860.4) centre (33580.2959, 18841.9) ccw
  arc A54 (33477.5, 18860.4) -> (33477.5, 18823.4) centre (33477.5, 18841.9) ccw
  line L505 (33477.5, 18183.4) -> (33580.2959, 18183.4)
  line L506 (33477.5, 18220.4) -> (33580.2959, 18220.4)
  arc A55 (33580.2959, 18183.4) -> (33580.2959, 18220.4) centre (33580.2959, 18201.9) ccw
  arc A56 (33477.5, 18220.4) -> (33477.5, 18183.4) centre (33477.5, 18201.9) ccw
  line L507 (33477.5, 17543.4) -> (33580.2959, 17543.4)
  line L508 (33477.5, 17580.4) -> (33580.2959, 17580.4)
  arc A57 (33580.2959, 17543.4) -> (33580.2959, 17580.4) centre (33580.2959, 17561.9) ccw
  arc A58 (33477.5, 17580.4) -> (33477.5, 17543.4) centre (33477.5, 17561.9) ccw
  line L509 (33393.529, 21328.4391) -> (33496.3249, 21328.4391)
  line L510 (33353, 14882.4) -> (33144.2114, 15119.9)
  line L511 (-80, 0) -> (0, 0) projected
  line L512 (33335, 14867.4) -> (33278.5113, 14816.9162)
  arc A59 (-95.715, -155.53) -> (-95.715, -205.53) centre (-95.715, -180.53) ccw
  arc A60 (634.2459, -205.53) -> (634.2459, -155.53) centre (634.2459, -180.53) ccw
  arc A61 (604.285, -155.53) -> (604.285, -205.53) centre (604.285, -180.53) ccw
  line L513 (269.2655, -155.53) -> (269.2655, 529.8236)
  line L514 (269.2655, 578.8236) -> (269.2655, 6518.16)
  line L515 (246.5579, -205.53) -> (291.973, -205.53)
  line L516 (246.5579, -155.53) -> (291.973, -155.53)
  arc A62 (291.973, -205.53) -> (291.973, -155.53) centre (291.973, -180.53) ccw
  arc A63 (246.5579, -155.53) -> (246.5579, -205.53) centre (246.5579, -180.53) ccw
  line L517 (-80.7345, -155.53) -> (-80.7345, 6518.16)
  line L518 (-95.715, -205.53) -> (-65.7541, -205.53)
  line L519 (-238.0845, 0) -> (762.4955, 0)
  line L520 (-385.5211, -25) -> (-263.0845, -25)
  line L521 (-385.5211, 25) -> (-263.0845, 25)
  arc A64 (-263.0845, -25) -> (-263.0845, 25) centre (-263.0845, 0) ccw
  line L522 (-95.715, -155.53) -> (-65.7541, -155.53)
  arc A65 (-385.5211, 25) -> (-385.5211, -25) centre (-385.5211, 0) ccw
  line L523 (619.2655, -155.53) -> (619.2655, 347.5)
  line L524 (-238.0845, 6400) -> (762.4955, 6400)
  line L525 (619.2655, 382.5) -> (619.2655, 6518.16)
  line L526 (604.285, -205.53) -> (634.2459, -205.53)
  line L527 (604.285, -155.53) -> (634.2459, -155.53)
  line L528 (-399.9791, 6375) -> (-263.0845, 6375)
  line L529 (-399.9791, 6425) -> (-263.0845, 6425)
  arc A66 (-263.0845, 6375) -> (-263.0845, 6425) centre (-263.0845, 6400) ccw
  arc A67 (-399.9791, 6425) -> (-399.9791, 6375) centre (-399.9791, 6400) ccw
  arc A68 (-65.7541, -205.53) -> (-65.7541, -155.53) centre (-65.7541, -180.53) ccw
  arc A69 (1058.1232, 6425) -> (1058.1232, 6375) centre (1058.1232, 6400) ccw
  arc A70 (1072.5812, 25) -> (1072.5812, -25) centre (1072.5812, 0) ccw
  line L530 (894.843, 2695) -> (884.843, 2695)
  line L531 (884.843, 2695) -> (889.843, 2720)
  line L532 (894.843, 2695) -> (889.843, 2720)
  line L533 (889.843, 4820) -> (889.843, 5170)
  line L534 (894.843, 1295) -> (884.843, 1295)
  line L535 (884.843, 1295) -> (889.843, 1320)
  line L536 (894.843, 1295) -> (889.843, 1320)
  line L537 (589.2655, 1320) -> (909.843, 1320)
  line L538 (894.843, 4795) -> (884.843, 4795)
  line L539 (884.843, 4795) -> (889.843, 4820)
  line L540 (894.843, 4795) -> (889.843, 4820)
  line L541 (589.2655, 4820) -> (909.843, 4820)
  line L542 (884.843, 4495) -> (894.843, 4495)
  line L543 (894.843, 4495) -> (889.843, 4470)
  line L544 (589.2655, 2720) -> (909.843, 2720)
  line L545 (884.843, 2395) -> (894.843, 2395)
  line L546 (894.843, 2395) -> (889.843, 2370)
  line L547 (884.843, 2395) -> (889.843, 2370)
  line L548 (884.843, 4495) -> (889.843, 4470)
  line L549 (589.2655, 4470) -> (909.843, 4470)
  line L550 (889.843, 4470) -> (889.843, 4820)
  line L551 (894.843, 4445) -> (884.843, 4445)
  line L552 (884.843, 4445) -> (889.843, 4470)
  line L553 (589.2655, 2370) -> (909.843, 2370)
  line L554 (884.843, 995) -> (894.843, 995)
  line L555 (894.843, 995) -> (889.843, 970)
  line L556 (884.843, 995) -> (889.843, 970)
  line L557 (894.843, 4445) -> (889.843, 4470)
  line L558 (589.2655, 4470) -> (909.843, 4470)
  line L559 (884.843, 4145) -> (894.843, 4145)
  line L560 (894.843, 4145) -> (889.843, 4120)
  line L561 (884.843, 4145) -> (889.843, 4120)
  line L562 (589.2655, 4120) -> (909.843, 4120)
  line L563 (889.843, 4120) -> (889.843, 4470)
  line L564 (889.843, 2370) -> (889.843, 2720)
  line L565 (894.843, 4095) -> (884.843, 4095)
  line L566 (884.843, 4095) -> (889.843, 4120)
  line L567 (894.843, 2345) -> (884.843, 2345)
  line L568 (884.843, 2345) -> (889.843, 2370)
  line L569 (894.843, 2345) -> (889.843, 2370)
  line L570 (589.2655, 970) -> (909.843, 970)
  line L571 (889.843, 970) -> (889.843, 1320)
  line L572 (589.2655, 2370) -> (909.843, 2370)
  line L573 (884.843, 2045) -> (894.843, 2045)
  line L574 (894.843, 2045) -> (889.843, 2020)
  line L575 (884.843, 2045) -> (889.843, 2020)
  line L576 (589.2655, 2020) -> (909.843, 2020)
  line L577 (889.843, 2020) -> (889.843, 2370)
  line L578 (894.843, 945) -> (884.843, 945)
  line L579 (589.2655, 3070) -> (909.843, 3070)
  line L580 (884.843, 945) -> (889.843, 970)
  line L581 (894.843, 1995) -> (884.843, 1995)
  line L582 (884.843, 1995) -> (889.843, 2020)
  line L583 (894.843, 1995) -> (889.843, 2020)
  line L584 (894.843, 5495) -> (889.843, 5520)
  line L585 (589.2655, 2020) -> (909.843, 2020)
  line L586 (884.843, 1695) -> (894.843, 1695)
  line L587 (894.843, 1695) -> (889.843, 1670)
  line L588 (884.843, 1695) -> (889.843, 1670)
  line L589 (894.843, 945) -> (889.843, 970)
  line L590 (589.2655, 970) -> (909.843, 970)
  line L591 (884.843, 645) -> (894.843, 645)
  line L592 (894.843, 645) -> (889.843, 620)
  line L593 (589.2655, 1670) -> (909.843, 1670)
  line L594 (889.843, 1670) -> (889.843, 2020)
  line L595 (884.843, 645) -> (889.843, 620)
  line L596 (589.2655, 620) -> (909.843, 620)
  line L597 (889.843, 620) -> (889.843, 970)
  line L598 (889.843, 0) -> (889.843, 620)
  line L599 (629.2655, 0) -> (909.843, 0)
  line L600 (884.843, 25) -> (889.843, 0)
  line L601 (894.843, 25) -> (889.843, 0)